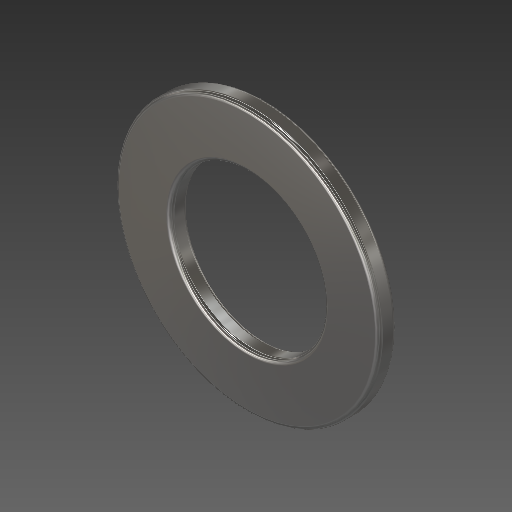
# Autodesk Inventor part: Arandela
Saved by Autodesk Inventor 2018 (Build 220112000, 112)
## iProperties
Created: 2016-06-28
Part Number: Arandela
Material: Steel
Document SubType Name: Modeling
Designer: YeseF
Density: 7.85 g/cm^3
Appearance: Steel - Polished
Author: YeseF
Autodesk Inventor part; units mm, degrees
ref_plane "YZ Plane" through (0, 0, 0) normal (1, 0, 0) x (0, 1, 0)
ref_plane "XZ Plane" through (0, 0, 0) normal (0, 1, 0) x (-1, 0, 0)
ref_plane "XY Plane" through (0, 0, 0) normal (0, 0, 1) x (1, 0, 0)
sketch "Sketch1" plane through (0, 0, 0) normal (0, 0, 1) x (1, 0, 0)
  circle A0 centre (0, 0) radius 14.5
  circle A1 centre (0, 0) radius 8.4
  dimension "d0" = 29
  dimension "d1" = 16.8
  constraints: 2 centre point, 2 coincident
  measures "d0" diameter of A0
  measures "d1" diameter of A1
extrude "Extrusion1" add sketch "Sketch1" along normal blind 2
fillet "Fillet1" radius 0.5 4 edges at (-14.5, 0, 2) (-14.5, 0, 0) (-8.4, 0, 2) (-8.4, 0, 0)
body "Solid1"
